Autodesk Fusion 360 part; units mm, degrees
(part 4 of 12)
  line L768 (-17.0192, 127.5167) -> (-12.6891, 125.0167)
  line L769 (-12.6891, 125.0167) -> (-8.359, 127.5167)
  line L770 (-8.359, 127.5167) -> (-8.359, 132.5167)
  line L771 (-8.359, 132.5167) -> (-12.6891, 135.0167)
  line L772 (-2.0289, 135.0167) -> (-6.359, 132.5167)
  line L773 (-6.359, 132.5167) -> (-6.359, 127.5167)
  line L774 (-6.359, 127.5167) -> (-2.0289, 125.0167)
  line L775 (-2.0289, 125.0167) -> (2.3013, 127.5167)
  line L776 (2.3013, 127.5167) -> (2.3013, 132.5167)
  line L777 (2.3013, 132.5167) -> (-2.0289, 135.0167)
  line L778 (8.6314, 135.0167) -> (4.3013, 132.5167)
  line L779 (4.3013, 132.5167) -> (4.3013, 127.5167)
  line L780 (4.3013, 127.5167) -> (8.6314, 125.0167)
  line L781 (8.6314, 125.0167) -> (12.9615, 127.5167)
  line L782 (12.9615, 127.5167) -> (12.9615, 132.5167)
  line L783 (12.9615, 132.5167) -> (8.6314, 135.0167)
  line L784 (19.2917, 135.0167) -> (14.9615, 132.5167)
  line L785 (14.9615, 132.5167) -> (14.9615, 127.5167)
  line L786 (14.9615, 127.5167) -> (19.2917, 125.0167)
  line L787 (19.2917, 125.0167) -> (23.6218, 127.5167)
  line L788 (23.6218, 127.5167) -> (23.6218, 132.5167)
  line L789 (23.6218, 132.5167) -> (19.2917, 135.0167)
  line L790 (29.9519, 135.0167) -> (25.6218, 132.5167)
  line L791 (25.6218, 132.5167) -> (25.6218, 127.5167)
  line L792 (25.6218, 127.5167) -> (29.9519, 125.0167)
  line L793 (29.9519, 125.0167) -> (34.282, 127.5167)
  line L794 (34.282, 127.5167) -> (34.282, 132.5167)
  line L795 (34.282, 132.5167) -> (29.9519, 135.0167)
  line L796 (40.6122, 135.0167) -> (36.282, 132.5167)
  line L797 (36.282, 132.5167) -> (36.282, 127.5167)
  line L798 (36.282, 127.5167) -> (40.6122, 125.0167)
  line L799 (40.6122, 125.0167) -> (44.9423, 127.5167)
  line L800 (44.9423, 127.5167) -> (44.9423, 132.5167)
  line L801 (44.9423, 132.5167) -> (40.6122, 135.0167)
  line L802 (-50, 144.2487) -> (-54.3301, 141.7487)
  line L803 (-54.3301, 141.7487) -> (-54.3301, 136.7487)
  line L804 (-54.3301, 136.7487) -> (-50, 134.2487)
  line L805 (-50, 134.2487) -> (-45.6699, 136.7487)
  line L806 (-45.6699, 136.7487) -> (-45.6699, 141.7487)
  line L807 (-45.6699, 141.7487) -> (-50, 144.2487)
  line L808 (-39.3397, 144.2487) -> (-43.6699, 141.7487)
  line L809 (-43.6699, 141.7487) -> (-43.6699, 136.7487)
  line L810 (-43.6699, 136.7487) -> (-39.3397, 134.2487)
  line L811 (-39.3397, 134.2487) -> (-35.0096, 136.7487)
  line L812 (-35.0096, 136.7487) -> (-35.0096, 141.7487)
  line L813 (-35.0096, 141.7487) -> (-39.3397, 144.2487)
  line L814 (-28.6795, 144.2487) -> (-33.0096, 141.7487)
  line L815 (-33.0096, 141.7487) -> (-33.0096, 136.7487)
  line L816 (-33.0096, 136.7487) -> (-28.6795, 134.2487)
  line L817 (-28.6795, 134.2487) -> (-24.3494, 136.7487)
  line L818 (-24.3494, 136.7487) -> (-24.3494, 141.7487)
  line L819 (-24.3494, 141.7487) -> (-28.6795, 144.2487)
  line L820 (-18.0192, 144.2487) -> (-22.3494, 141.7487)
  line L821 (-22.3494, 141.7487) -> (-22.3494, 136.7487)
  line L822 (-22.3494, 136.7487) -> (-18.0192, 134.2487)
  line L823 (-18.0192, 134.2487) -> (-13.6891, 136.7487)
  line L824 (-13.6891, 136.7487) -> (-13.6891, 141.7487)
  line L825 (-13.6891, 141.7487) -> (-18.0192, 144.2487)
  line L826 (-7.359, 144.2487) -> (-11.6891, 141.7487)
  line L827 (-11.6891, 141.7487) -> (-11.6891, 136.7487)
  line L828 (-11.6891, 136.7487) -> (-7.359, 134.2487)
  line L829 (-7.359, 134.2487) -> (-3.0289, 136.7487)
  line L830 (-3.0289, 136.7487) -> (-3.0289, 141.7487)
  line L831 (-3.0289, 141.7487) -> (-7.359, 144.2487)
  line L832 (3.3013, 144.2487) -> (-1.0289, 141.7487)
  line L833 (-1.0289, 141.7487) -> (-1.0289, 136.7487)
  line L834 (-1.0289, 136.7487) -> (3.3013, 134.2487)
  line L835 (3.3013, 134.2487) -> (7.6314, 136.7487)
  line L836 (7.6314, 136.7487) -> (7.6314, 141.7487)
  line L837 (7.6314, 141.7487) -> (3.3013, 144.2487)
  line L838 (13.9615, 144.2487) -> (9.6314, 141.7487)
  line L839 (9.6314, 141.7487) -> (9.6314, 136.7487)
  line L840 (9.6314, 136.7487) -> (13.9615, 134.2487)
  line L841 (13.9615, 134.2487) -> (18.2917, 136.7487)
  line L842 (18.2917, 136.7487) -> (18.2917, 141.7487)
  line L843 (18.2917, 141.7487) -> (13.9615, 144.2487)
  line L844 (24.6218, 144.2487) -> (20.2917, 141.7487)
  line L845 (20.2917, 141.7487) -> (20.2917, 136.7487)
  line L846 (20.2917, 136.7487) -> (24.6218, 134.2487)
  line L847 (24.6218, 134.2487) -> (28.9519, 136.7487)
  line L848 (28.9519, 136.7487) -> (28.9519, 141.7487)
  line L849 (28.9519, 141.7487) -> (24.6218, 144.2487)
  line L850 (35.282, 144.2487) -> (30.9519, 141.7487)
  line L851 (30.9519, 141.7487) -> (30.9519, 136.7487)
  line L852 (30.9519, 136.7487) -> (35.282, 134.2487)
  line L853 (35.282, 134.2487) -> (39.6122, 136.7487)
  line L854 (39.6122, 136.7487) -> (39.6122, 141.7487)
  line L855 (39.6122, 141.7487) -> (35.282, 144.2487)
  line L856 (45.9423, 144.2487) -> (41.6122, 141.7487)
  line L857 (41.6122, 141.7487) -> (41.6122, 136.7487)
  line L858 (41.6122, 136.7487) -> (45.9423, 134.2487)
  line L859 (45.9423, 134.2487) -> (50.2724, 136.7487)
  line L860 (50.2724, 136.7487) -> (50.2724, 141.7487)
  line L861 (50.2724, 141.7487) -> (45.9423, 144.2487)
  line L862 (-44.6699, 153.4808) -> (-49, 150.9808)
  line L863 (-49, 150.9808) -> (-49, 145.9808)
  line L864 (-49, 145.9808) -> (-44.6699, 143.4808)
  line L865 (-44.6699, 143.4808) -> (-40.3397, 145.9808)
  line L866 (-40.3397, 145.9808) -> (-40.3397, 150.9808)
  line L867 (-40.3397, 150.9808) -> (-44.6699, 153.4808)
  line L868 (-34.0096, 153.4808) -> (-38.3397, 150.9808)
  line L869 (-38.3397, 150.9808) -> (-38.3397, 145.9808)
  line L870 (-38.3397, 145.9808) -> (-34.0096, 143.4808)
  line L871 (-34.0096, 143.4808) -> (-29.6795, 145.9808)
  line L872 (-29.6795, 145.9808) -> (-29.6795, 150.9808)
  line L873 (-29.6795, 150.9808) -> (-34.0096, 153.4808)
  line L874 (-23.3494, 153.4808) -> (-27.6795, 150.9808)
  line L875 (-27.6795, 150.9808) -> (-27.6795, 145.9808)
  line L876 (-27.6795, 145.9808) -> (-23.3494, 143.4808)
  line L877 (-23.3494, 143.4808) -> (-19.0192, 145.9808)
  line L878 (-19.0192, 145.9808) -> (-19.0192, 150.9808)
  line L879 (-19.0192, 150.9808) -> (-23.3494, 153.4808)
  line L880 (-12.6891, 153.4808) -> (-17.0192, 150.9808)
  line L881 (-17.0192, 150.9808) -> (-17.0192, 145.9808)
  line L882 (-17.0192, 145.9808) -> (-12.6891, 143.4808)
  line L883 (-12.6891, 143.4808) -> (-8.359, 145.9808)
  line L884 (-8.359, 145.9808) -> (-8.359, 150.9808)
  line L885 (-8.359, 150.9808) -> (-12.6891, 153.4808)
  line L886 (-2.0289, 153.4808) -> (-6.359, 150.9808)
  line L887 (-6.359, 150.9808) -> (-6.359, 145.9808)
  line L888 (-6.359, 145.9808) -> (-2.0289, 143.4808)
  line L889 (-2.0289, 143.4808) -> (2.3013, 145.9808)
  line L890 (2.3013, 145.9808) -> (2.3013, 150.9808)
  line L891 (2.3013, 150.9808) -> (-2.0289, 153.4808)
  line L892 (8.6314, 153.4808) -> (4.3013, 150.9808)
  line L893 (4.3013, 150.9808) -> (4.3013, 145.9808)
  line L894 (4.3013, 145.9808) -> (8.6314, 143.4808)
  line L895 (8.6314, 143.4808) -> (12.9615, 145.9808)
  line L896 (12.9615, 145.9808) -> (12.9615, 150.9808)
  line L897 (12.9615, 150.9808) -> (8.6314, 153.4808)
  line L898 (19.2917, 153.4808) -> (14.9615, 150.9808)
  line L899 (14.9615, 150.9808) -> (14.9615, 145.9808)
  line L900 (14.9615, 145.9808) -> (19.2917, 143.4808)
  line L901 (19.2917, 143.4808) -> (23.6218, 145.9808)
  line L902 (23.6218, 145.9808) -> (23.6218, 150.9808)
  line L903 (23.6218, 150.9808) -> (19.2917, 153.4808)
  line L904 (29.9519, 153.4808) -> (25.6218, 150.9808)
  line L905 (25.6218, 150.9808) -> (25.6218, 145.9808)
  line L906 (25.6218, 145.9808) -> (29.9519, 143.4808)
  line L907 (29.9519, 143.4808) -> (34.282, 145.9808)
  line L908 (34.282, 145.9808) -> (34.282, 150.9808)
  line L909 (34.282, 150.9808) -> (29.9519, 153.4808)
  line L910 (40.6122, 153.4808) -> (36.282, 150.9808)
  line L911 (36.282, 150.9808) -> (36.282, 145.9808)
  line L912 (36.282, 145.9808) -> (40.6122, 143.4808)
  line L913 (40.6122, 143.4808) -> (44.9423, 145.9808)
  line L914 (44.9423, 145.9808) -> (44.9423, 150.9808)
  line L915 (44.9423, 150.9808) -> (40.6122, 153.4808)
  line L916 (-50, 162.7128) -> (-54.3301, 160.2128)
  line L917 (-54.3301, 160.2128) -> (-54.3301, 155.2128)
  line L918 (-54.3301, 155.2128) -> (-50, 152.7128)
  line L919 (-50, 152.7128) -> (-45.6699, 155.2128)
  line L920 (-45.6699, 155.2128) -> (-45.6699, 160.2128)
  line L921 (-45.6699, 160.2128) -> (-50, 162.7128)
  line L922 (-39.3397, 162.7128) -> (-43.6699, 160.2128)
  line L923 (-43.6699, 160.2128) -> (-43.6699, 155.2128)
  line L924 (-43.6699, 155.2128) -> (-39.3397, 152.7128)
  line L925 (-39.3397, 152.7128) -> (-35.0096, 155.2128)
  line L926 (-35.0096, 155.2128) -> (-35.0096, 160.2128)
  line L927 (-35.0096, 160.2128) -> (-39.3397, 162.7128)
  line L928 (-28.6795, 162.7128) -> (-33.0096, 160.2128)
  line L929 (-33.0096, 160.2128) -> (-33.0096, 155.2128)
  line L930 (-33.0096, 155.2128) -> (-28.6795, 152.7128)
  line L931 (-28.6795, 152.7128) -> (-24.3494, 155.2128)
  line L932 (-24.3494, 155.2128) -> (-24.3494, 160.2128)
  line L933 (-24.3494, 160.2128) -> (-28.6795, 162.7128)
  line L934 (-18.0192, 162.7128) -> (-22.3494, 160.2128)
  line L935 (-22.3494, 160.2128) -> (-22.3494, 155.2128)
  line L936 (-22.3494, 155.2128) -> (-18.0192, 152.7128)
  line L937 (-18.0192, 152.7128) -> (-13.6891, 155.2128)
  line L938 (-13.6891, 155.2128) -> (-13.6891, 160.2128)
  line L939 (-13.6891, 160.2128) -> (-18.0192, 162.7128)
  line L940 (-7.359, 162.7128) -> (-11.6891, 160.2128)
  line L941 (-11.6891, 160.2128) -> (-11.6891, 155.2128)
  line L942 (-11.6891, 155.2128) -> (-7.359, 152.7128)
  line L943 (-7.359, 152.7128) -> (-3.0289, 155.2128)
  line L944 (-3.0289, 155.2128) -> (-3.0289, 160.2128)
  line L945 (-3.0289, 160.2128) -> (-7.359, 162.7128)
  line L946 (3.3013, 162.7128) -> (-1.0289, 160.2128)
  line L947 (-1.0289, 160.2128) -> (-1.0289, 155.2128)
  line L948 (-1.0289, 155.2128) -> (3.3013, 152.7128)
  line L949 (3.3013, 152.7128) -> (7.6314, 155.2128)
  line L950 (7.6314, 155.2128) -> (7.6314, 160.2128)
  line L951 (7.6314, 160.2128) -> (3.3013, 162.7128)
  line L952 (13.9615, 162.7128) -> (9.6314, 160.2128)
  line L953 (9.6314, 160.2128) -> (9.6314, 155.2128)
  line L954 (9.6314, 155.2128) -> (13.9615, 152.7128)
  line L955 (13.9615, 152.7128) -> (18.2917, 155.2128)
  line L956 (18.2917, 155.2128) -> (18.2917, 160.2128)
  line L957 (18.2917, 160.2128) -> (13.9615, 162.7128)
  line L958 (24.6218, 162.7128) -> (20.2917, 160.2128)
  line L959 (20.2917, 160.2128) -> (20.2917, 155.2128)
  line L960 (20.2917, 155.2128) -> (24.6218, 152.7128)
  line L961 (24.6218, 152.7128) -> (28.9519, 155.2128)
  line L962 (28.9519, 155.2128) -> (28.9519, 160.2128)
  line L963 (28.9519, 160.2128) -> (24.6218, 162.7128)
  line L964 (35.282, 162.7128) -> (30.9519, 160.2128)
  line L965 (30.9519, 160.2128) -> (30.9519, 155.2128)
  line L966 (30.9519, 155.2128) -> (35.282, 152.7128)
  line L967 (35.282, 152.7128) -> (39.6122, 155.2128)
  line L968 (39.6122, 155.2128) -> (39.6122, 160.2128)
  line L969 (39.6122, 160.2128) -> (35.282, 162.7128)
  line L970 (45.9423, 162.7128) -> (41.6122, 160.2128)
  line L971 (41.6122, 160.2128) -> (41.6122, 155.2128)
  line L972 (41.6122, 155.2128) -> (45.9423, 152.7128)
  line L973 (45.9423, 152.7128) -> (50.2724, 155.2128)
  line L974 (50.2724, 155.2128) -> (50.2724, 160.2128)
  line L975 (50.2724, 160.2128) -> (45.9423, 162.7128)
  line L976 (-44.6699, 171.9449) -> (-49, 169.4449)
  line L977 (-49, 169.4449) -> (-49, 164.4449)
  line L978 (-49, 164.4449) -> (-44.6699, 161.9449)
  line L979 (-44.6699, 161.9449) -> (-40.3397, 164.4449)
  line L980 (-40.3397, 164.4449) -> (-40.3397, 169.4449)
  line L981 (-40.3397, 169.4449) -> (-44.6699, 171.9449)
  line L982 (-34.0096, 171.9449) -> (-38.3397, 169.4449)
  line L983 (-38.3397, 169.4449) -> (-38.3397, 164.4449)
  line L984 (-38.3397, 164.4449) -> (-34.0096, 161.9449)
  line L985 (-34.0096, 161.9449) -> (-29.6795, 164.4449)
  line L986 (-29.6795, 164.4449) -> (-29.6795, 169.4449)
  line L987 (-29.6795, 169.4449) -> (-34.0096, 171.9449)
  line L988 (-23.3494, 171.9449) -> (-27.6795, 169.4449)
  line L989 (-27.6795, 169.4449) -> (-27.6795, 164.4449)
  line L990 (-27.6795, 164.4449) -> (-23.3494, 161.9449)
  line L991 (-23.3494, 161.9449) -> (-19.0192, 164.4449)
  line L992 (-19.0192, 164.4449) -> (-19.0192, 169.4449)
  line L993 (-19.0192, 169.4449) -> (-23.3494, 171.9449)
  line L994 (-12.6891, 171.9449) -> (-17.0192, 169.4449)
  line L995 (-17.0192, 169.4449) -> (-17.0192, 164.4449)
  line L996 (-17.0192, 164.4449) -> (-12.6891, 161.9449)
  line L997 (-12.6891, 161.9449) -> (-8.359, 164.4449)
  line L998 (-8.359, 164.4449) -> (-8.359, 169.4449)
  line L999 (-8.359, 169.4449) -> (-12.6891, 171.9449)
  line L1000 (-2.0289, 171.9449) -> (-6.359, 169.4449)
  line L1001 (-6.359, 169.4449) -> (-6.359, 164.4449)
  line L1002 (-6.359, 164.4449) -> (-2.0289, 161.9449)
  line L1003 (-2.0289, 161.9449) -> (2.3013, 164.4449)
  line L1004 (2.3013, 164.4449) -> (2.3013, 169.4449)
  line L1005 (2.3013, 169.4449) -> (-2.0289, 171.9449)
  line L1006 (8.6314, 171.9449) -> (4.3013, 169.4449)
  line L1007 (4.3013, 169.4449) -> (4.3013, 164.4449)
  line L1008 (4.3013, 164.4449) -> (8.6314, 161.9449)
  line L1009 (8.6314, 161.9449) -> (12.9615, 164.4449)
  line L1010 (12.9615, 164.4449) -> (12.9615, 169.4449)
  line L1011 (12.9615, 169.4449) -> (8.6314, 171.9449)
  line L1012 (19.2917, 171.9449) -> (14.9615, 169.4449)
  line L1013 (14.9615, 169.4449) -> (14.9615, 164.4449)
  line L1014 (14.9615, 164.4449) -> (19.2917, 161.9449)
  line L1015 (19.2917, 161.9449) -> (23.6218, 164.4449)
  line L1016 (23.6218, 164.4449) -> (23.6218, 169.4449)
  line L1017 (23.6218, 169.4449) -> (19.2917, 171.9449)
  line L1018 (29.9519, 171.9449) -> (25.6218, 169.4449)
  line L1019 (25.6218, 169.4449) -> (25.6218, 164.4449)
  line L1020 (25.6218, 164.4449) -> (29.9519, 161.9449)
  line L1021 (29.9519, 161.9449) -> (34.282, 164.4449)
  line L1022 (34.282, 164.4449) -> (34.282, 169.4449)
  line L1023 (34.282, 169.4449) -> (29.9519, 171.9449)
  line L1024 (40.6122, 171.9449) -> (36.282, 169.4449)
  line L1025 (36.282, 169.4449) -> (36.282, 164.4449)
  line L1026 (36.282, 164.4449) -> (40.6122, 161.9449)
  line L1027 (40.6122, 161.9449) -> (44.9423, 164.4449)
  line L1028 (44.9423, 164.4449) -> (44.9423, 169.4449)
  line L1029 (44.9423, 169.4449) -> (40.6122, 171.9449)
  line L1030 (-50, 181.1769) -> (-54.3301, 178.6769)
  line L1031 (-54.3301, 178.6769) -> (-54.3301, 173.6769)
  line L1032 (-54.3301, 173.6769) -> (-50, 171.1769)
  line L1033 (-50, 171.1769) -> (-45.6699, 173.6769)
  line L1034 (-45.6699, 173.6769) -> (-45.6699, 178.6769)
  line L1035 (-45.6699, 178.6769) -> (-50, 181.1769)
  line L1036 (-39.3397, 181.1769) -> (-43.6699, 178.6769)
  line L1037 (-43.6699, 178.6769) -> (-43.6699, 173.6769)
  line L1038 (-43.6699, 173.6769) -> (-39.3397, 171.1769)
  line L1039 (-39.3397, 171.1769) -> (-35.0096, 173.6769)
  line L1040 (-35.0096, 173.6769) -> (-35.0096, 178.6769)
  line L1041 (-35.0096, 178.6769) -> (-39.3397, 181.1769)
  line L1042 (-28.6795, 181.1769) -> (-33.0096, 178.6769)
  line L1043 (-33.0096, 178.6769) -> (-33.0096, 173.6769)
  line L1044 (-33.0096, 173.6769) -> (-28.6795, 171.1769)
  line L1045 (-28.6795, 171.1769) -> (-24.3494, 173.6769)
  line L1046 (-24.3494, 173.6769) -> (-24.3494, 178.6769)
  line L1047 (-24.3494, 178.6769) -> (-28.6795, 181.1769)
  line L1048 (-18.0192, 181.1769) -> (-22.3494, 178.6769)
  line L1049 (-22.3494, 178.6769) -> (-22.3494, 173.6769)
  line L1050 (-22.3494, 173.6769) -> (-18.0192, 171.1769)
  line L1051 (-18.0192, 171.1769) -> (-13.6891, 173.6769)
  line L1052 (-13.6891, 173.6769) -> (-13.6891, 178.6769)
  line L1053 (-13.6891, 178.6769) -> (-18.0192, 181.1769)
  line L1054 (-7.359, 181.1769) -> (-11.6891, 178.6769)
  line L1055 (-11.6891, 178.6769) -> (-11.6891, 173.6769)
  line L1056 (-11.6891, 173.6769) -> (-7.359, 171.1769)
  line L1057 (-7.359, 171.1769) -> (-3.0289, 173.6769)
  line L1058 (-3.0289, 173.6769) -> (-3.0289, 178.6769)
  line L1059 (-3.0289, 178.6769) -> (-7.359, 181.1769)
  line L1060 (3.3013, 181.1769) -> (-1.0289, 178.6769)
  line L1061 (-1.0289, 178.6769) -> (-1.0289, 173.6769)
  line L1062 (-1.0289, 173.6769) -> (3.3013, 171.1769)
  line L1063 (3.3013, 171.1769) -> (7.6314, 173.6769)
  line L1064 (7.6314, 173.6769) -> (7.6314, 178.6769)
  line L1065 (7.6314, 178.6769) -> (3.3013, 181.1769)
  line L1066 (13.9615, 181.1769) -> (9.6314, 178.6769)
  line L1067 (9.6314, 178.6769) -> (9.6314, 173.6769)
  line L1068 (9.6314, 173.6769) -> (13.9615, 171.1769)
  line L1069 (13.9615, 171.1769) -> (18.2917, 173.6769)
  line L1070 (18.2917, 173.6769) -> (18.2917, 178.6769)
  line L1071 (18.2917, 178.6769) -> (13.9615, 181.1769)
  line L1072 (24.6218, 181.1769) -> (20.2917, 178.6769)
  line L1073 (20.2917, 178.6769) -> (20.2917, 173.6769)
  line L1074 (20.2917, 173.6769) -> (24.6218, 171.1769)
  line L1075 (24.6218, 171.1769) -> (28.9519, 173.6769)
  line L1076 (28.9519, 173.6769) -> (28.9519, 178.6769)
  line L1077 (28.9519, 178.6769) -> (24.6218, 181.1769)
  line L1078 (35.282, 181.1769) -> (30.9519, 178.6769)
  line L1079 (30.9519, 178.6769) -> (30.9519, 173.6769)
  line L1080 (30.9519, 173.6769) -> (35.282, 171.1769)
  line L1081 (35.282, 171.1769) -> (39.6122, 173.6769)
  line L1082 (39.6122, 173.6769) -> (39.6122, 178.6769)
  line L1083 (39.6122, 178.6769) -> (35.282, 181.1769)
  line L1084 (45.9423, 181.1769) -> (41.6122, 178.6769)
  line L1085 (41.6122, 178.6769) -> (41.6122, 173.6769)
  line L1086 (41.6122, 173.6769) -> (45.9423, 171.1769)
  line L1087 (45.9423, 171.1769) -> (50.2724, 173.6769)
  line L1088 (50.2724, 173.6769) -> (50.2724, 178.6769)
  line L1089 (50.2724, 178.6769) -> (45.9423, 181.1769)
  line L1090 (-44.6699, 190.409) -> (-49, 187.909)
  line L1091 (-49, 187.909) -> (-49, 182.909)
  line L1092 (-49, 182.909) -> (-44.6699, 180.409)
  line L1093 (-44.6699, 180.409) -> (-40.3397, 182.909)
  line L1094 (-40.3397, 182.909) -> (-40.3397, 187.909)
  line L1095 (-40.3397, 187.909) -> (-44.6699, 190.409)
  line L1096 (-34.0096, 190.409) -> (-38.3397, 187.909)
  line L1097 (-38.3397, 187.909) -> (-38.3397, 182.909)
  line L1098 (-38.3397, 182.909) -> (-34.0096, 180.409)
  line L1099 (-34.0096, 180.409) -> (-29.6795, 182.909)
  line L1100 (-29.6795, 182.909) -> (-29.6795, 187.909)
  line L1101 (-29.6795, 187.909) -> (-34.0096, 190.409)
  line L1102 (-23.3494, 190.409) -> (-27.6795, 187.909)
  line L1103 (-27.6795, 187.909) -> (-27.6795, 182.909)
  line L1104 (-27.6795, 182.909) -> (-23.3494, 180.409)
  line L1105 (-23.3494, 180.409) -> (-19.0192, 182.909)
  line L1106 (-19.0192, 182.909) -> (-19.0192, 187.909)
  line L1107 (-19.0192, 187.909) -> (-23.3494, 190.409)
  line L1108 (-12.6891, 190.409) -> (-17.0192, 187.909)
  line L1109 (-17.0192, 187.909) -> (-17.0192, 182.909)
  line L1110 (-17.0192, 182.909) -> (-12.6891, 180.409)
  line L1111 (-12.6891, 180.409) -> (-8.359, 182.909)
  line L1112 (-8.359, 182.909) -> (-8.359, 187.909)
  line L1113 (-8.359, 187.909) -> (-12.6891, 190.409)
  line L1114 (-2.0289, 190.409) -> (-6.359, 187.909)
  line L1115 (-6.359, 187.909) -> (-6.359, 182.909)
  line L1116 (-6.359, 182.909) -> (-2.0289, 180.409)
  line L1117 (-2.0289, 180.409) -> (2.3013, 182.909)
  line L1118 (2.3013, 182.909) -> (2.3013, 187.909)
  line L1119 (2.3013, 187.909) -> (-2.0289, 190.409)
  line L1120 (8.6314, 190.409) -> (4.3013, 187.909)
  line L1121 (4.3013, 187.909) -> (4.3013, 182.909)
  line L1122 (4.3013, 182.909) -> (8.6314, 180.409)
  line L1123 (8.6314, 180.409) -> (12.9615, 182.909)
  line L1124 (12.9615, 182.909) -> (12.9615, 187.909)
  line L1125 (12.9615, 187.909) -> (8.6314, 190.409)
  line L1126 (19.2917, 190.409) -> (14.9615, 187.909)
  line L1127 (14.9615, 187.909) -> (14.9615, 182.909)
  line L1128 (14.9615, 182.909) -> (19.2917, 180.409)
  line L1129 (19.2917, 180.409) -> (23.6218, 182.909)
  line L1130 (23.6218, 182.909) -> (23.6218, 187.909)
  line L1131 (23.6218, 187.909) -> (19.2917, 190.409)
  line L1132 (29.9519, 190.409) -> (25.6218, 187.909)
  line L1133 (25.6218, 187.909) -> (25.6218, 182.909)
  line L1134 (25.6218, 182.909) -> (29.9519, 180.409)
  line L1135 (29.9519, 180.409) -> (34.282, 182.909)
  line L1136 (34.282, 182.909) -> (34.282, 187.909)
  line L1137 (34.282, 187.909) -> (29.9519, 190.409)
  line L1138 (40.6122, 190.409) -> (36.282, 187.909)
  line L1139 (36.282, 187.909) -> (36.282, 182.909)
  line L1140 (36.282, 182.909) -> (40.6122, 180.409)
  line L1141 (40.6122, 180.409) -> (44.9423, 182.909)
  line L1142 (44.9423, 182.909) -> (44.9423, 187.909)
  line L1143 (44.9423, 187.909) -> (40.6122, 190.409)
  line L1144 (-50, 199.641) -> (-54.3301, 197.141)
  line L1145 (-54.3301, 197.141) -> (-54.3301, 192.141)
  line L1146 (-54.3301, 192.141) -> (-50, 189.641)
  line L1147 (-50, 189.641) -> (-45.6699, 192.141)
  line L1148 (-45.6699, 192.141) -> (-45.6699, 197.141)
  line L1149 (-45.6699, 197.141) -> (-50, 199.641)
  line L1150 (-39.3397, 199.641) -> (-43.6699, 197.141)
  line L1151 (-43.6699, 197.141) -> (-43.6699, 192.141)
  line L1152 (-43.6699, 192.141) -> (-39.3397, 189.641)
  line L1153 (-39.3397, 189.641) -> (-35.0096, 192.141)
  line L1154 (-35.0096, 192.141) -> (-35.0096, 197.141)
  line L1155 (-35.0096, 197.141) -> (-39.3397, 199.641)
  line L1156 (-28.6795, 199.641) -> (-33.0096, 197.141)
  line L1157 (-33.0096, 197.141) -> (-33.0096, 192.141)
  line L1158 (-33.0096, 192.141) -> (-28.6795, 189.641)
  line L1159 (-28.6795, 189.641) -> (-24.3494, 192.141)
  line L1160 (-24.3494, 192.141) -> (-24.3494, 197.141)
  line L1161 (-24.3494, 197.141) -> (-28.6795, 199.641)
  line L1162 (-18.0192, 199.641) -> (-22.3494, 197.141)
  line L1163 (-22.3494, 197.141) -> (-22.3494, 192.141)
  line L1164 (-22.3494, 192.141) -> (-18.0192, 189.641)
  line L1165 (-18.0192, 189.641) -> (-13.6891, 192.141)
  line L1166 (-13.6891, 192.141) -> (-13.6891, 197.141)
  line L1167 (-13.6891, 197.141) -> (-18.0192, 199.641)
  line L1168 (-7.359, 199.641) -> (-11.6891, 197.141)
  line L1169 (-11.6891, 197.141) -> (-11.6891, 192.141)
  line L1170 (-11.6891, 192.141) -> (-7.359, 189.641)
  line L1171 (-7.359, 189.641) -> (-3.0289, 192.141)
  line L1172 (-3.0289, 192.141) -> (-3.0289, 197.141)
  line L1173 (-3.0289, 197.141) -> (-7.359, 199.641)
  line L1174 (3.3013, 199.641) -> (-1.0289, 197.141)
  line L1175 (-1.0289, 197.141) -> (-1.0289, 192.141)
  line L1176 (-1.0289, 192.141) -> (3.3013, 189.641)
  line L1177 (3.3013, 189.641) -> (7.6314, 192.141)
  line L1178 (7.6314, 192.141) -> (7.6314, 197.141)
  line L1179 (7.6314, 197.141) -> (3.3013, 199.641)
  line L1180 (13.9615, 199.641) -> (9.6314, 197.141)
  line L1181 (9.6314, 197.141) -> (9.6314, 192.141)
  line L1182 (9.6314, 192.141) -> (13.9615, 189.641)
  line L1183 (13.9615, 189.641) -> (18.2917, 192.141)
  line L1184 (18.2917, 192.141) -> (18.2917, 197.141)
  line L1185 (18.2917, 197.141) -> (13.9615, 199.641)
  line L1186 (24.6218, 199.641) -> (20.2917, 197.141)
  line L1187 (20.2917, 197.141) -> (20.2917, 192.141)
  line L1188 (20.2917, 192.141) -> (24.6218, 189.641)
  line L1189 (24.6218, 189.641) -> (28.9519, 192.141)
  line L1190 (28.9519, 192.141) -> (28.9519, 197.141)
  line L1191 (28.9519, 197.141) -> (24.6218, 199.641)
  line L1192 (35.282, 199.641) -> (30.9519, 197.141)
  line L1193 (30.9519, 197.141) -> (30.9519, 192.141)
  line L1194 (30.9519, 192.141) -> (35.282, 189.641)
  line L1195 (35.282, 189.641) -> (39.6122, 192.141)
  line L1196 (39.6122, 192.141) -> (39.6122, 197.141)
  line L1197 (39.6122, 197.141) -> (35.282, 199.641)
  line L1198 (45.9423, 199.641) -> (41.6122, 197.141)
  line L1199 (41.6122, 197.141) -> (41.6122, 192.141)
  line L1200 (41.6122, 192.141) -> (45.9423, 189.641)
  line L1201 (45.9423, 189.641) -> (50.2724, 192.141)
  line L1202 (50.2724, 192.141) -> (50.2724, 197.141)
  line L1203 (50.2724, 197.141) -> (45.9423, 199.641)
  line L1204 (-44.6699, 208.8731) -> (-49, 206.3731)
  line L1205 (-49, 206.3731) -> (-49, 201.3731)
  line L1206 (-49, 201.3731) -> (-44.6699, 198.8731)
  line L1207 (-44.6699, 198.8731) -> (-40.3397, 201.3731)
  line L1208 (-40.3397, 201.3731) -> (-40.3397, 206.3731)
  line L1209 (-40.3397, 206.3731) -> (-44.6699, 208.8731)
  line L1210 (-34.0096, 208.8731) -> (-38.3397, 206.3731)
  line L1211 (-38.3397, 206.3731) -> (-38.3397, 201.3731)
  line L1212 (-38.3397, 201.3731) -> (-34.0096, 198.8731)
  line L1213 (-34.0096, 198.8731) -> (-29.6795, 201.3731)
  line L1214 (-29.6795, 201.3731) -> (-29.6795, 206.3731)
  line L1215 (-29.6795, 206.3731) -> (-34.0096, 208.8731)
  line L1216 (-23.3494, 208.8731) -> (-27.6795, 206.3731)
  line L1217 (-27.6795, 206.3731) -> (-27.6795, 201.3731)
  line L1218 (-27.6795, 201.3731) -> (-23.3494, 198.8731)
  line L1219 (-23.3494, 198.8731) -> (-19.0192, 201.3731)
  line L1220 (-19.0192, 201.3731) -> (-19.0192, 206.3731)
  line L1221 (-19.0192, 206.3731) -> (-23.3494, 208.8731)
  line L1222 (-12.6891, 208.8731) -> (-17.0192, 206.3731)
  line L1223 (-17.0192, 206.3731) -> (-17.0192, 201.3731)
  line L1224 (-17.0192, 201.3731) -> (-12.6891, 198.8731)
  line L1225 (-12.6891, 198.8731) -> (-8.359, 201.3731)
  line L1226 (-8.359, 201.3731) -> (-8.359, 206.3731)
  line L1227 (-8.359, 206.3731) -> (-12.6891, 208.8731)
  line L1228 (-2.0289, 208.8731) -> (-6.359, 206.3731)
  line L1229 (-6.359, 206.3731) -> (-6.359, 201.3731)
  line L1230 (-6.359, 201.3731) -> (-2.0289, 198.8731)
  line L1231 (-2.0289, 198.8731) -> (2.3013, 201.3731)
  line L1232 (2.3013, 201.3731) -> (2.3013, 206.3731)
  line L1233 (2.3013, 206.3731) -> (-2.0289, 208.8731)
  line L1234 (8.6314, 208.8731) -> (4.3013, 206.3731)
  line L1235 (4.3013, 206.3731) -> (4.3013, 201.3731)
  line L1236 (4.3013, 201.3731) -> (8.6314, 198.8731)
  line L1237 (8.6314, 198.8731) -> (12.9615, 201.3731)
  line L1238 (12.9615, 201.3731) -> (12.9615, 206.3731)
  line L1239 (12.9615, 206.3731) -> (8.6314, 208.8731)
  line L1240 (19.2917, 208.8731) -> (14.9615, 206.3731)
  line L1241 (14.9615, 206.3731) -> (14.9615, 201.3731)
  line L1242 (14.9615, 201.3731) -> (19.2917, 198.8731)
  line L1243 (19.2917, 198.8731) -> (23.6218, 201.3731)
  line L1244 (23.6218, 201.3731) -> (23.6218, 206.3731)
  line L1245 (23.6218, 206.3731) -> (19.2917, 208.8731)
  line L1246 (29.9519, 208.8731) -> (25.6218, 206.3731)
  line L1247 (25.6218, 206.3731) -> (25.6218, 201.3731)
  line L1248 (25.6218, 201.3731) -> (29.9519, 198.8731)
  line L1249 (29.9519, 198.8731) -> (34.282, 201.3731)
  line L1250 (34.282, 201.3731) -> (34.282, 206.3731)
  line L1251 (34.282, 206.3731) -> (29.9519, 208.8731)
  line L1252 (40.6122, 208.8731) -> (36.282, 206.3731)
  line L1253 (36.282, 206.3731) -> (36.282, 201.3731)
  line L1254 (36.282, 201.3731) -> (40.6122, 198.8731)
  line L1255 (40.6122, 198.8731) -> (44.9423, 201.3731)
  line L1256 (44.9423, 201.3731) -> (44.9423, 206.3731)
  line L1257 (44.9423, 206.3731) -> (40.6122, 208.8731)
  line L1258 (-50, 218.1051) -> (-54.3301, 215.6051)
  line L1259 (-54.3301, 215.6051) -> (-54.3301, 210.6051)
  line L1260 (-54.3301, 210.6051) -> (-50, 208.1051)
  line L1261 (-50, 208.1051) -> (-45.6699, 210.6051)
  line L1262 (-45.6699, 210.6051) -> (-45.6699, 215.6051)
  line L1263 (-45.6699, 215.6051) -> (-50, 218.1051)
  line L1264 (-39.3397, 218.1051) -> (-43.6699, 215.6051)
  line L1265 (-43.6699, 215.6051) -> (-43.6699, 210.6051)
  line L1266 (-43.6699, 210.6051) -> (-39.3397, 208.1051)
  line L1267 (-39.3397, 208.1051) -> (-35.0096, 210.6051)
  line L1268 (-35.0096, 210.6051) -> (-35.0096, 215.6051)
  line L1269 (-35.0096, 215.6051) -> (-39.3397, 218.1051)
  line L1270 (-28.6795, 218.1051) -> (-33.0096, 215.6051)
  line L1271 (-33.0096, 215.6051) -> (-33.0096, 210.6051)
  line L1272 (-33.0096, 210.6051) -> (-28.6795, 208.1051)
  line L1273 (-28.6795, 208.1051) -> (-24.3494, 210.6051)
  line L1274 (-24.3494, 210.6051) -> (-24.3494, 215.6051)
  line L1275 (-24.3494, 215.6051) -> (-28.6795, 218.1051)
  line L1276 (-18.0192, 218.1051) -> (-22.3494, 215.6051)
  line L1277 (-22.3494, 215.6051) -> (-22.3494, 210.6051)
  line L1278 (-22.3494, 210.6051) -> (-18.0192, 208.1051)
  line L1279 (-18.0192, 208.1051) -> (-13.6891, 210.6051)
  line L1280 (-13.6891, 210.6051) -> (-13.6891, 215.6051)
  line L1281 (-13.6891, 215.6051) -> (-18.0192, 218.1051)
  line L1282 (-7.359, 218.1051) -> (-11.6891, 215.6051)
  line L1283 (-11.6891, 215.6051) -> (-11.6891, 210.6051)
  line L1284 (-11.6891, 210.6051) -> (-7.359, 208.1051)
  line L1285 (-7.359, 208.1051) -> (-3.0289, 210.6051)
  line L1286 (-3.0289, 210.6051) -> (-3.0289, 215.6051)
  line L1287 (-3.0289, 215.6051) -> (-7.359, 218.1051)
  line L1288 (3.3013, 218.1051) -> (-1.0289, 215.6051)
  line L1289 (-1.0289, 215.6051) -> (-1.0289, 210.6051)
  line L1290 (-1.0289, 210.6051) -> (3.3013, 208.1051)
  line L1291 (3.3013, 208.1051) -> (7.6314, 210.6051)
  line L1292 (7.6314, 210.6051) -> (7.6314, 215.6051)
  line L1293 (7.6314, 215.6051) -> (3.3013, 218.1051)
  line L1294 (13.9615, 218.1051) -> (9.6314, 215.6051)
  line L1295 (9.6314, 215.6051) -> (9.6314, 210.6051)
  line L1296 (9.6314, 210.6051) -> (13.9615, 208.1051)
  line L1297 (13.9615, 208.1051) -> (18.2917, 210.6051)
  line L1298 (18.2917, 210.6051) -> (18.2917, 215.6051)
  line L1299 (18.2917, 215.6051) -> (13.9615, 218.1051)
  line L1300 (24.6218, 218.1051) -> (20.2917, 215.6051)
  line L1301 (20.2917, 215.6051) -> (20.2917, 210.6051)
  line L1302 (20.2917, 210.6051) -> (24.6218, 208.1051)
  line L1303 (24.6218, 208.1051) -> (28.9519, 210.6051)
  line L1304 (28.9519, 210.6051) -> (28.9519, 215.6051)
  line L1305 (28.9519, 215.6051) -> (24.6218, 218.1051)
  line L1306 (35.282, 218.1051) -> (30.9519, 215.6051)
  line L1307 (30.9519, 215.6051) -> (30.9519, 210.6051)
  line L1308 (30.9519, 210.6051) -> (35.282, 208.1051)
  line L1309 (35.282, 208.1051) -> (39.6122, 210.6051)
  line L1310 (39.6122, 210.6051) -> (39.6122, 215.6051)
  line L1311 (39.6122, 215.6051) -> (35.282, 218.1051)
  line L1312 (45.9423, 218.1051) -> (41.6122, 215.6051)
  line L1313 (41.6122, 215.6051) -> (41.6122, 210.6051)
  line L1314 (41.6122, 210.6051) -> (45.9423, 208.1051)
  line L1315 (45.9423, 208.1051) -> (50.2724, 210.6051)
  line L1316 (50.2724, 210.6051) -> (50.2724, 215.6051)
  line L1317 (50.2724, 215.6051) -> (45.9423, 218.1051)
  line L1318 (-44.6699, 227.3372) -> (-49, 224.8372)
  line L1319 (-49, 224.8372) -> (-49, 219.8372)
  line L1320 (-49, 219.8372) -> (-44.6699, 217.3372)
  line L1321 (-44.6699, 217.3372) -> (-40.3397, 219.8372)
  line L1322 (-40.3397, 219.8372) -> (-40.3397, 224.8372)
  line L1323 (-40.3397, 224.8372) -> (-44.6699, 227.3372)
  line L1324 (-34.0096, 227.3372) -> (-38.3397, 224.8372)
  line L1325 (-38.3397, 224.8372) -> (-38.3397, 219.8372)
  line L1326 (-38.3397, 219.8372) -> (-34.0096, 217.3372)
  line L1327 (-34.0096, 217.3372) -> (-29.6795, 219.8372)
  line L1328 (-29.6795, 219.8372) -> (-29.6795, 224.8372)
  line L1329 (-29.6795, 224.8372) -> (-34.0096, 227.3372)
  line L1330 (-23.3494, 227.3372) -> (-27.6795, 224.8372)
  line L1331 (-27.6795, 224.8372) -> (-27.6795, 219.8372)
  line L1332 (-27.6795, 219.8372) -> (-23.3494, 217.3372)
  line L1333 (-23.3494, 217.3372) -> (-19.0192, 219.8372)
  line L1334 (-19.0192, 219.8372) -> (-19.0192, 224.8372)
  line L1335 (-19.0192, 224.8372) -> (-23.3494, 227.3372)
  line L1336 (-12.6891, 227.3372) -> (-17.0192, 224.8372)
  line L1337 (-17.0192, 224.8372) -> (-17.0192, 219.8372)
  line L1338 (-17.0192, 219.8372) -> (-12.6891, 217.3372)
  line L1339 (-12.6891, 217.3372) -> (-8.359, 219.8372)
  line L1340 (-8.359, 219.8372) -> (-8.359, 224.8372)
  line L1341 (-8.359, 224.8372) -> (-12.6891, 227.3372)
  line L1342 (-2.0289, 227.3372) -> (-6.359, 224.8372)
  line L1343 (-6.359, 224.8372) -> (-6.359, 219.8372)
  line L1344 (-6.359, 219.8372) -> (-2.0289, 217.3372)
  line L1345 (-2.0289, 217.3372) -> (2.3013, 219.8372)
  line L1346 (2.3013, 219.8372) -> (2.3013, 224.8372)
  line L1347 (2.3013, 224.8372) -> (-2.0289, 227.3372)
  line L1348 (8.6314, 227.3372) -> (4.3013, 224.8372)
  line L1349 (4.3013, 224.8372) -> (4.3013, 219.8372)
  line L1350 (4.3013, 219.8372) -> (8.6314, 217.3372)
  line L1351 (8.6314, 217.3372) -> (12.9615, 219.8372)
  line L1352 (12.9615, 219.8372) -> (12.9615, 224.8372)
  line L1353 (12.9615, 224.8372) -> (8.6314, 227.3372)
  line L1354 (19.2917, 227.3372) -> (14.9615, 224.8372)
  line L1355 (14.9615, 224.8372) -> (14.9615, 219.8372)
  line L1356 (14.9615, 219.8372) -> (19.2917, 217.3372)
  line L1357 (19.2917, 217.3372) -> (23.6218, 219.8372)
  line L1358 (23.6218, 219.8372) -> (23.6218, 224.8372)
  line L1359 (23.6218, 224.8372) -> (19.2917, 227.3372)
  line L1360 (29.9519, 227.3372) -> (25.6218, 224.8372)
  line L1361 (25.6218, 224.8372) -> (25.6218, 219.8372)
  line L1362 (25.6218, 219.8372) -> (29.9519, 217.3372)
  line L1363 (29.9519, 217.3372) -> (34.282, 219.8372)
  line L1364 (34.282, 219.8372) -> (34.282, 224.8372)
  line L1365 (34.282, 224.8372) -> (29.9519, 227.3372)
  line L1366 (40.6122, 227.3372) -> (36.282, 224.8372)
  line L1367 (36.282, 224.8372) -> (36.282, 219.8372)
  line L1368 (36.282, 219.8372) -> (40.6122, 217.3372)
  line L1369 (40.6122, 217.3372) -> (44.9423, 219.8372)
  line L1370 (44.9423, 219.8372) -> (44.9423, 224.8372)
  line L1371 (44.9423, 224.8372) -> (40.6122, 227.3372)
  line L1372 (-50, 236.5692) -> (-54.3301, 234.0692)
  line L1373 (-54.3301, 234.0692) -> (-54.3301, 229.0692)
  line L1374 (-54.3301, 229.0692) -> (-50, 226.5692)
  line L1375 (-50, 226.5692) -> (-45.6699, 229.0692)
  line L1376 (-45.6699, 229.0692) -> (-45.6699, 234.0692)
  line L1377 (-45.6699, 234.0692) -> (-50, 236.5692)
  line L1378 (-39.3397, 236.5692) -> (-43.6699, 234.0692)
  line L1379 (-43.6699, 234.0692) -> (-43.6699, 229.0692)
  line L1380 (-43.6699, 229.0692) -> (-39.3397, 226.5692)
  line L1381 (-39.3397, 226.5692) -> (-35.0096, 229.0692)
  line L1382 (-35.0096, 229.0692) -> (-35.0096, 234.0692)
  line L1383 (-35.0096, 234.0692) -> (-39.3397, 236.5692)
  line L1384 (-28.6795, 236.5692) -> (-33.0096, 234.0692)
  line L1385 (-33.0096, 234.0692) -> (-33.0096, 229.0692)
  line L1386 (-33.0096, 229.0692) -> (-28.6795, 226.5692)
  line L1387 (-28.6795, 226.5692) -> (-24.3494, 229.0692)
  line L1388 (-24.3494, 229.0692) -> (-24.3494, 234.0692)
  line L1389 (-24.3494, 234.0692) -> (-28.6795, 236.5692)
  line L1390 (-18.0192, 236.5692) -> (-22.3494, 234.0692)
  line L1391 (-22.3494, 234.0692) -> (-22.3494, 229.0692)
  line L1392 (-22.3494, 229.0692) -> (-18.0192, 226.5692)
  line L1393 (-18.0192, 226.5692) -> (-13.6891, 229.0692)
  line L1394 (-13.6891, 229.0692) -> (-13.6891, 234.0692)
  line L1395 (-13.6891, 234.0692) -> (-18.0192, 236.5692)
  line L1396 (-7.359, 236.5692) -> (-11.6891, 234.0692)
  line L1397 (-11.6891, 234.0692) -> (-11.6891, 229.0692)
  line L1398 (-11.6891, 229.0692) -> (-7.359, 226.5692)
  line L1399 (-7.359, 226.5692) -> (-3.0289, 229.0692)
  line L1400 (-3.0289, 229.0692) -> (-3.0289, 234.0692)
  line L1401 (-3.0289, 234.0692) -> (-7.359, 236.5692)
  line L1402 (3.3013, 236.5692) -> (-1.0289, 234.0692)
  line L1403 (-1.0289, 234.0692) -> (-1.0289, 229.0692)
  line L1404 (-1.0289, 229.0692) -> (3.3013, 226.5692)
  line L1405 (3.3013, 226.5692) -> (7.6314, 229.0692)
  line L1406 (7.6314, 229.0692) -> (7.6314, 234.0692)
  line L1407 (7.6314, 234.0692) -> (3.3013, 236.5692)
  line L1408 (13.9615, 236.5692) -> (9.6314, 234.0692)
  line L1409 (9.6314, 234.0692) -> (9.6314, 229.0692)
  line L1410 (9.6314, 229.0692) -> (13.9615, 226.5692)
  line L1411 (13.9615, 226.5692) -> (18.2917, 229.0692)
  line L1412 (18.2917, 229.0692) -> (18.2917, 234.0692)
  line L1413 (18.2917, 234.0692) -> (13.9615, 236.5692)
  line L1414 (24.6218, 236.5692) -> (20.2917, 234.0692)
  line L1415 (20.2917, 234.0692) -> (20.2917, 229.0692)
  line L1416 (20.2917, 229.0692) -> (24.6218, 226.5692)
  line L1417 (24.6218, 226.5692) -> (28.9519, 229.0692)
  line L1418 (28.9519, 229.0692) -> (28.9519, 234.0692)
  line L1419 (28.9519, 234.0692) -> (24.6218, 236.5692)
  line L1420 (35.282, 236.5692) -> (30.9519, 234.0692)
  line L1421 (30.9519, 234.0692) -> (30.9519, 229.0692)
  line L1422 (30.9519, 229.0692) -> (35.282, 226.5692)
  line L1423 (35.282, 226.5692) -> (39.6122, 229.0692)
  line L1424 (39.6122, 229.0692) -> (39.6122, 234.0692)
  line L1425 (39.6122, 234.0692) -> (35.282, 236.5692)
  line L1426 (45.9423, 236.5692) -> (41.6122, 234.0692)
  line L1427 (41.6122, 234.0692) -> (41.6122, 229.0692)
  line L1428 (41.6122, 229.0692) -> (45.9423, 226.5692)
  line L1429 (45.9423, 226.5692) -> (50.2724, 229.0692)
  line L1430 (50.2724, 229.0692) -> (50.2724, 234.0692)
  line L1431 (50.2724, 234.0692) -> (45.9423, 236.5692)
extrude "拉伸5" cut sketch "草图26" against normal blind 4 contours L4 L5 L6 L7 L8 L9 | L10 L11 L12 L13 L14 L15 | L16 L17 L18 L19 L20 L21 | L22 L23 L24 L25 L26 L27 | L28 L29 L30 L31 L32 L33 | L34 L35 L36 L37 L38 L39 | L40 L41 L42 L43 L44 L45 | L46 L47 L48 L49 L50 L51 | L52 L53 L54 L55 L56 L57 | L58 L59 L60 L61 L62 L63 | L64 L65 L66 L67 L68 L69 | L70 L71 L72 L73 L74 L75 | L76 L77 L78 L79 L80 L81 | L82 L83 L84 L85 L86 L87 | L88 L89 L90 L91 L92 L93 | L94 L95 L96 L97 L98 L99 | L100 L101 L102 L103 L104 L105 | L106 L107 L108 L109 L110 L111 | L112 L113 L114 L115 L116 L117 | L118 L119 L120 L121 L122 L123 | L124 L125 L126 L127 L128 L129 | L130 L131 L132 L133 L134 L135 | L136 L137 L138 L139 L140 L141 | L142 L143 L144 L145 L146 L147 | L148 L149 L150 L151 L152 L153 | L154 L155 L156 L157 L158 L159 | L160 L161 L162 L163 L164 L165 | L166 L167 L168 L169 L170 L171 | L172 L173 L174 L175 L176 L177 | L178 L179 L180 L181 L182 L183 | L184 L185 L186 L187 L188 L189 | L190 L191 L192 L193 L194 L195 | L196 L197 L198 L199 L200 L201 | L202 L203 L204 L205 L206 L207 | L208 L209 L210 L211 L212 L213 | L214 L215 L216 L217 L218 L219 | L220 L221 L222 L223 L224 L225 | L226 L227 L228 L229 L230 L231 | L232 L233 L234 L235 L236 L237 | L238 L239 L240 L241 L242 L243 | L244 L245 L246 L247 L248 L249 | L250 L251 L252 L253 L254 L255 | L256 L257 L258 L259 L260 L261 | L262 L263 L264 L265 L266 L267 | L268 L269 L270 L271 L272 L273 | L274 L275 L276 L277 L278 L279 | L280 L281 L282 L283 L284 L285 | L286 L287 L288 L289 L290 L291 | L292 L293 L294 L295 L296 L297 | L298 L299 L300 L301 L302 L303 | L304 L305 L306 L307 L308 L309 | L310 L311 L312 L313 L314 L315 | L316 L317 L318 L319 L320 L321 | L322 L323 L324 L325 L326 L327 | L328 L329 L330 L331 L332 L333 | L334 L335 L336 L337 L338 L339 | L340 L341 L342 L343 L344 L345 | L346 L347 L348 L349 L350 L351 | L352 L353 L354 L355 L356 L357 | L358 L359 L360 L361 L362 L363 | L364 L365 L366 L367 L368 L369 | L370 L371 L372 L373 L374 L375 | L376 L377 L378 L379 L380 L381 | L382 L383 L384 L385 L386 L387 | L388 L389 L390 L391 L392 L393 | L394 L395 L396 L397 L398 L399 | L400 L401 L402 L403 L404 L405 | L406 L407 L408 L409 L410 L411 | L412 L413 L414 L415 L416 L417 | L418 L419 L420 L421 L422 L423 | L424 L425 L426 L427 L428 L429 | L430 L431 L432 L433 L434 L435 | L436 L437 L438 L439 L440 L441 | L442 L443 L444 L445 L446 L447 | L448 L449 L450 L451 L452 L453 | L454 L455 L456 L457 L458 L459 | L460 L461 L462 L463 L464 L465 | L466 L467 L468 L469 L470 L471 | L472 L473 L474 L475 L476 L477 | L478 L479 L480 L481 L482 L483 | L484 L485 L486 L487 L488 L489 | L490 L491 L492 L493 L494 L495 | L496 L497 L498 L499 L500 L501 | L502 L503 L504 L505 L506 L507 | L508 L509 L510 L511 L512 L513 | L514 L515 L516 L517 L518 L519 | L520 L521 L522 L523 L524 L525 | L526 L527 L528 L529 L530 L531 | L532 L533 L534 L535 L536 L537 | L538 L539 L540 L541 L542 L543 | L544 L545 L546 L547 L548 L549 | L550 L551 L552 L553 L554 L555 | L556 L557 L558 L559 L560 L561 | L562 L563 L564 L565 L566 L567 | L568 L569 L570 L571 L572 L573 | L574 L575 L576 L577 L578 L579 | L580 L581 L582 L583 L584 L585 | L586 L587 L588 L589 L590 L591 | L592 L593 L594 L595 L596 L597 | L598 L599 L600 L601 L602 L603 | L604 L605 L606 L607 L608 L609 | L610 L611 L612 L613 L614 L615 | L616 L617 L618 L619 L620 L621 | L622 L623 L624 L625 L626 L627 | L628 L629 L630 L631 L632 L633 | L634 L635 L636 L637 L638 L639 | L640 L641 L642 L643 L644 L645 | L646 L647 L648 L649 L650 L651 | L652 L653 L654 L655 L656 L657 | L658 L659 L660 L661 L662 L663 | L664 L665 L666 L667 L668 L669 | L670 L671 L672 L673 L674 L675 | L676 L677 L678 L679 L680 L681 | L682 L683 L684 L685 L686 L687 | L688 L689 L690 L691 L692 L693 | L694 L695 L696 L697 L698 L699 | L700 L701 L702 L703 L704 L705 | L706 L707 L708 L709 L710 L711 | L712 L713 L714 L715 L716 L717 | L718 L719 L720 L721 L722 L723 | L724 L725 L726 L727 L728 L729 | L730 L731 L732 L733 L734 L735 | L736 L737 L738 L739 L740 L741 | L742 L743 L744 L745 L746 L747 | L748 L749 L750 L751 L752 L753 | L754 L755 L756 L757 L758 L759 | L760 L761 L762 L763 L764 L765 | L766 L767 L768 L769 L770 L771 | L772 L773 L774 L775 L776 L777 | L778 L779 L780 L781 L782 L783 | L784 L785 L786 L787 L788 L789 | L790 L791 L792 L793 L794 L795 | L796 L797 L798 L799 L800 L801 | L802 L803 L804 L805 L806 L807 | L808 L809 L810 L811 L812 L813 | L814 L815 L816 L817 L818 L819 | L820 L821 L822 L823 L824 L825 | L826 L827 L828 L829 L830 L831 | L832 L833 L834 L835 L836 L837 | L838 L839 L840 L841 L842 L843 | L844 L845 L846 L847 L848 L849 | L850 L851 L852 L853 L854 L855 | L856 L857 L858 L859 L860 L861 | L862 L863 L864 L865 L866 L867 | L868 L869 L870 L871 L872 L873 | L874 L875 L876 L877 L878 L879 | L880 L881 L882 L883 L884 L885 | L886 L887 L888 L889 L890 L891 | L892 L893 L894 L895 L896 L897 | L898 L899 L900 L901 L902 L903 | L904 L905 L906 L907 L908 L909 | L910 L911 L912 L913 L914 L915 | L916 L917 L918 L919 L920 L921 | L922 L923 L924 L925 L926 L927 | L928 L929 L930 L931 L932 L933 | L934 L935 L936 L937 L938 L939 | L940 L941 L942 L943 L944 L945 | L946 L947 L948 L949 L950 L951 | L952 L953 L954 L955 L956 L957 | L958 L959 L960 L961 L962 L963 | L964 L965 L966 L967 L968 L969 | L970 L971 L972 L973 L974 L975 | L976 L977 L978 L979 L980 L981 | L982 L983 L984 L985 L986 L987 | L988 L989 L990 L991 L992 L993 | L994 L995 L996 L997 L998 L999 | L1000 L1001 L1002 L1003 L1004 L1005 | L1006 L1007 L1008 L1009 L1010 L1011 | L1012 L1013 L1014 L1015 L1016 L1017 | L1018 L1019 L1020 L1021 L1022 L1023 | L1024 L1025 L1026 L1027 L1028 L1029 | L1030 L1031 L1032 L1033 L1034 L1035 | L1036 L1037 L1038 L1039 L1040 L1041 | L1042 L1043 L1044 L1045 L1046 L1047 | L1048 L1049 L1050 L1051 L1052 L1053 | L1054 L1055 L1056 L1057 L1058 L1059 | L1060 L1061 L1062 L1063 L1064 L1065 | L1066 L1067 L1068 L1069 L1070 L1071 | L1072 L1073 L1074 L1075 L1076 L1077 | L1078 L1079 L1080 L1081 L1082 L1083 | L1084 L1085 L1086 L1087 L1088 L1089 | L1090 L1091 L1092 L1093 L1094 L1095 | L1096 L1097 L1098 L1099 L1100 L1101 | L1102 L1103 L1104 L1105 L1106 L1107 | L1108 L1109 L1110 L1111 L1112 L1113 | L1114 L1115 L1116 L1117 L1118 L1119 | L1120 L1121 L1122 L1123 L1124 L1125 | L1126 L1127 L1128 L1129 L1130 L1131 | L1132 L1133 L1134 L1135 L1136 L1137 | L1138 L1139 L1140 L1141 L1142 L1143 | L1144 L1145 L1146 L1147 L1148 L1149 | L1150 L1151 L1152 L1153 L1154 L1155 | L1156 L1157 L1158 L1159 L1160 L1161 | L1162 L1163 L1164 L1165 L1166 L1167 | L1168 L1169 L1170 L1171 L1172 L1173 | L1174 L1175 L1176 L1177 L1178 L1179 | L1180 L1181 L1182 L1183 L1184 L1185 | L1186 L1187 L1188 L1189 L1190 L1191 | L1192 L1193 L1194 L1195 L1196 L1197 | L1198 L1199 L1200 L1201 L1202 L1203 | L1204 L1205 L1206 L1207 L1208 L1209 | L1210 L1211 L1212 L1213 L1214 L1215 | L1216 L1217 L1218 L1219 L1220 L1221 | L1222 L1223 L1224 L1225 L1226 L1227 | L1228 L1229 L1230 L1231 L1232 L1233 | L1234 L1235 L1236 L1237 L1238 L1239 | L1240 L1241 L1242 L1243 L1244 L1245 | L1246 L1247 L1248 L1249 L1250 L1251 | L1252 L1253 L1254 L1255 L1256 L1257 | L1258 L1259 L1260 L1261 L1262 L1263 | L1264 L1265 L1266 L1267 L1268 L1269 | L1270 L1271 L1272 L1273 L1274 L1275 | L1276 L1277 L1278 L1279 L1280 L1281 | L1282 L1283 L1284 L1285 L1286 L1287 | L1288 L1289 L1290 L1291 L1292 L1293 | L1294 L1295 L1296 L1297 L1298 L1299 | L1300 L1301 L1302 L1303 L1304 L1305 | L1306 L1307 L1308 L1309 L1310 L1311 | L1312 L1313 L1314 L1315 L1316 L1317 | L1318 L1319 L1320 L1321 L1322 L1323 | L1324 L1325 L1326 L1327 L1328 L1329 | L1330 L1331 L1332 L1333 L1334 L1335 | L1336 L1337 L1338 L1339 L1340 L1341 | L1342 L1343 L1344 L1345 L1346 L1347 | L1348 L1349 L1350 L1351 L1352 L1353 | L1354 L1355 L1356 L1357 L1358 L1359 | L1360 L1361 L1362 L1363 L1364 L1365 | L1366 L1367 L1368 L1369 L1370 L1371 | L1372 L1373 L1374 L1375 L1376 L1377 | L1378 L1379 L1380 L1381 L1382 L1383 | L1384 L1385 L1386 L1387 L1388 L1389 | L1390 L1391 L1392 L1393 L1394 L1395 | L1396 L1397 L1398 L1399 L1400 L1401 | L1402 L1403 L1404 L1405 L1406 L1407 | L1408 L1409 L1410 L1411 L1412 L1413 | L1414 L1415 L1416 L1417 L1418 L1419 | L1420 L1421 L1422 L1423 L1424 L1425 | L1426 L1427 L1428 L1429 L1430 L1431